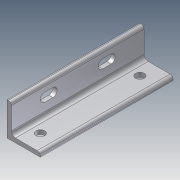
# Autodesk Inventor part: GE-12102
Saved by Autodesk Inventor 2012 (Build 160160000, 160)
## iProperties
Created: 2011-08-08
Part Number: GE-12102
Document SubType Name: Modeling
Designer: mcyr
Density: 1 g/cm^3
Description: Angle, Sensor Bracket
Mass: 14.6108 g
Surface Area: 101.713 cm^2
Volume: 14.6108 cm^3
Material: Default
Title: Angle, Sensor Bracket
Author: mcyr
Autodesk Inventor part; units mm, degrees
ref_plane "YZ Plane" through (0, 0, 0) normal (1, 0, 0) x (0, 1, 0)
ref_plane "XZ Plane" through (0, 0, 0) normal (0, 1, 0) x (-1, 0, 0)
ref_plane "XY Plane" through (0, 0, 0) normal (0, 0, 1) x (1, 0, 0)
sketch "Sketch1" plane through (0, 0, 0) normal (0, 0, 1) x (1, 0, 0)
  line L0 (0, 25.4) -> (0, 0)
  line L1 (0, 0) -> (25.4, 0)
  line L2 (25.4, 0) -> (25.4, 3.175)
  line L3 (25.4, 3.175) -> (3.175, 3.175)
  line L4 (3.175, 3.175) -> (3.175, 25.4)
  line L5 (3.175, 25.4) -> (0, 25.4)
  dimension "d0" = 25.4
  dimension "d1" = 25.4
  dimension "d2" = 3.175
  dimension "d3" = 3.175
  constraints: 12 end point, 4 parallel, 1 perpendicular, 1 vertical
  measures "d0" distance of L0.start L0.end
  measures "d1" distance of L0.end L1.end
  measures "d2" distance of L1.end L2.end
  measures "d3" distance of L4.end L0.start
extrude "Extrusion1" add sketch "Sketch1" along normal blind 101.6
fillet "Fillet1" radius 3.175 1 edges at (3.175, 3.175, 50.8)
hole "Hole1" at (12.7, 3.175, 88.9) direction (0, -1, 0) diameter 6.731 end through all
pattern_linear "Rectangular Pattern1" count 2 spacing 76.2 along (0, 0, -1) of "Hole1"
fillet "Fillet3" radius 2.3876 2 edges at (3.175, 25.4, 50.8) (25.4, 3.175, 50.8)
sketch "Sketch2" plane through (3.175, 6.35, 101.6) normal (1, 0, 0) x (0, 0, -1)
  line L0 (0, 16.6624) -> (0, 0) projected
  line L1 (101.6, 16.6624) -> (101.6, 0) projected
  arc A0 (25.4, 12.8905) -> (25.4, 6.1595) centre (25.4, 9.525) ccw
  arc A1 (31.75, 6.1595) -> (31.75, 12.8905) centre (31.75, 9.525) ccw
  arc A2 (69.85, 12.8905) -> (69.85, 6.1595) centre (69.85, 9.525) ccw
  arc A3 (76.2, 6.1595) -> (76.2, 12.8905) centre (76.2, 9.525) ccw
  line L2 (25.4, 12.8905) -> (31.75, 12.8905)
  line L3 (31.75, 6.1595) -> (25.4, 6.1595)
  line L4 (69.85, 12.8905) -> (76.2, 12.8905)
  line L5 (76.2, 6.1595) -> (69.85, 6.1595)
  line L6 (101.6, -6.35) -> (0, -6.35) projected
  dimension "d21" = 6.731
  dimension "d22" = 6.35
  dimension "d23" = 6.35
  dimension "d24" = 15.875
  dimension "d25" = 15.875
  dimension "d26" = 25.4
  dimension "d27" = 25.4
  constraints: 8 end point, 8 point on circle, 8 tangent, 4 centre point, 3 equal radius, 1 horizontal, 1 parallel
  measures "d21" diameter of A0
  measures "d22" distance of A1.centre A0.centre
  measures "d23" distance of A3.centre A2.centre
  measures "d24" distance from line of A0.centre L6
  measures "d25" distance from line of A2.centre L6
  measures "d26" distance from line of A0.centre L0
  measures "d27" distance from line of L1 A3.centre
extrude "Extrusion2" cut sketch "Sketch2" against normal blind 25.4
body "Solid1"
